Autodesk Fusion 360 part; units mm, degrees
(part 4 of 6)
  line L1889 (94.173, 59.875) -> (98.4623, 59.875)
  line L1890 (93.1162, 65.9119) -> (93.971, 59.875)
  line L1891 (98.4284, 66.8385) -> (97.7686, 66.2013)
  line L1892 (93.9606, 61.375) -> (94.173, 59.875)
  line L1893 (93.1277, 66.1876) -> (97.4664, 66.1876)
  line L1894 (98.4003, 67.0365) -> (97.5043, 67.9621)
  line L1895 (91.4702, 66.8375) -> (92.2202, 66.8375)
  line L1896 (99.1784, 66.8385) -> (98.4284, 66.8385)
  arc A278 (92.3951, 60.3049) -> (92.8902, 59.875) centre (92.8902, 60.375) ccw
  line L1897 (92.1918, 67.0375) -> (91.4418, 67.0375)
  line L1898 (96.4494, 74) -> (96.6618, 72.5)
  arc A279 (98.2252, 73.5701) -> (97.7301, 74) centre (97.7301, 73.5) ccw
  line L1899 (91.4418, 67.0375) -> (90.456, 74)
  line L1900 (92.3834, 72.5) -> (92.171, 74)
  line L1901 (98.1643, 74) -> (99.1503, 67.0365)
  line L1902 (92.3894, 66.9502) -> (93.1277, 66.1876)
  line L1903 (91.971, 74) -> (92.8648, 67.6874)
  line L1904 (98.23, 66.9249) -> (97.4917, 67.6876)
  line L1905 (97.5043, 67.9621) -> (96.6494, 74)
  line L1906 (92.171, 74) -> (96.4494, 74)
  line L1907 (97.4917, 67.6876) -> (93.1529, 67.6876)
  line L1908 (96.6494, 74) -> (98.1643, 74)
  line L1909 (92.8648, 67.6874) -> (92.1918, 67.0375)
  line L1910 (109.3698, 72.5) -> (105.0914, 72.5)
  line L1911 (104.679, 74) -> (103.164, 74)
  arc A280 (112.2965, 59.875) -> (112.7916, 60.4451) centre (112.2965, 60.375) ccw
  circle A281 centre (103.164, 60.75) radius 0.875
  line L1912 (104.9282, 66.8375) -> (105.8242, 65.9119)
  line L1913 (111.3723, 59.875) -> (112.8723, 59.875)
  line L1914 (110.9579, 61.375) -> (106.6686, 61.375)
  line L1915 (105.8609, 67.6876) -> (105.0974, 66.9502)
  line L1916 (106.679, 59.875) -> (105.164, 59.875)
  line L1917 (105.164, 59.875) -> (104.1782, 66.8375)
  line L1918 (110.4766, 66.2013) -> (111.3723, 59.875)
  line L1919 (111.1703, 59.875) -> (110.9579, 61.375)
  line L1920 (110.1744, 66.1876) -> (110.938, 66.9249)
  line L1921 (111.8583, 67.0365) -> (111.1083, 67.0365)
  line L1922 (112.8723, 59.875) -> (111.8864, 66.8385)
  arc A282 (103.7398, 74) -> (103.2447, 73.4299) centre (103.7398, 73.5) ccw
  line L1923 (106.881, 59.875) -> (111.1703, 59.875)
  line L1924 (105.8242, 65.9119) -> (106.679, 59.875)
  line L1925 (111.1364, 66.8385) -> (110.4766, 66.2013)
  line L1926 (106.6686, 61.375) -> (106.881, 59.875)
  line L1927 (105.8357, 66.1876) -> (110.1744, 66.1876)
  line L1928 (111.1083, 67.0365) -> (110.2123, 67.9621)
  line L1929 (104.1782, 66.8375) -> (104.9282, 66.8375)
  line L1930 (111.8864, 66.8385) -> (111.1364, 66.8385)
  arc A283 (105.1031, 60.3049) -> (105.5982, 59.875) centre (105.5982, 60.375) ccw
  line L1931 (104.8998, 67.0375) -> (104.1498, 67.0375)
  line L1932 (109.1574, 74) -> (109.3698, 72.5)
  arc A284 (110.9332, 73.5701) -> (110.4381, 74) centre (110.4381, 73.5) ccw
  line L1933 (104.1498, 67.0375) -> (103.164, 74)
  line L1934 (105.0914, 72.5) -> (104.879, 74)
  line L1935 (110.8723, 74) -> (111.8583, 67.0365)
  line L1936 (105.0974, 66.9502) -> (105.8357, 66.1876)
  line L1937 (104.679, 74) -> (105.5728, 67.6874)
  line L1938 (110.938, 66.9249) -> (110.1997, 67.6876)
  line L1939 (110.2123, 67.9621) -> (109.3574, 74)
  line L1940 (104.879, 74) -> (109.1574, 74)
  line L1941 (110.1997, 67.6876) -> (105.8609, 67.6876)
  line L1942 (109.3574, 74) -> (110.8723, 74)
  line L1943 (105.5728, 67.6874) -> (104.8998, 67.0375)
  line L1944 (122.0778, 72.5) -> (117.7994, 72.5)
  line L1945 (117.387, 74) -> (115.872, 74)
  arc A285 (125.0045, 59.875) -> (125.4996, 60.4451) centre (125.0045, 60.375) ccw
  circle A286 centre (115.872, 60.75) radius 0.875
  line L1946 (117.6362, 66.8375) -> (118.5322, 65.9119)
  line L1947 (124.0803, 59.875) -> (125.5803, 59.875)
  line L1948 (123.6659, 61.375) -> (119.3766, 61.375)
  line L1949 (118.5689, 67.6876) -> (117.8054, 66.9502)
  line L1950 (119.387, 59.875) -> (117.872, 59.875)
  line L1951 (117.872, 59.875) -> (116.8862, 66.8375)
  line L1952 (123.1846, 66.2013) -> (124.0803, 59.875)
  line L1953 (123.8783, 59.875) -> (123.6659, 61.375)
  line L1954 (122.8824, 66.1876) -> (123.646, 66.9249)
  line L1955 (124.5663, 67.0365) -> (123.8163, 67.0365)
  line L1956 (125.5803, 59.875) -> (124.5944, 66.8385)
  arc A287 (116.4478, 74) -> (115.9527, 73.4299) centre (116.4478, 73.5) ccw
  line L1957 (119.589, 59.875) -> (123.8783, 59.875)
  line L1958 (118.5322, 65.9119) -> (119.387, 59.875)
  line L1959 (123.8444, 66.8385) -> (123.1846, 66.2013)
  line L1960 (119.3766, 61.375) -> (119.589, 59.875)
  line L1961 (118.5437, 66.1876) -> (122.8824, 66.1876)
  line L1962 (123.8163, 67.0365) -> (122.9203, 67.9621)
  line L1963 (116.8862, 66.8375) -> (117.6362, 66.8375)
  line L1964 (124.5944, 66.8385) -> (123.8444, 66.8385)
  arc A288 (117.8111, 60.3049) -> (118.3062, 59.875) centre (118.3062, 60.375) ccw
  line L1965 (117.6078, 67.0375) -> (116.8578, 67.0375)
  line L1966 (121.8654, 74) -> (122.0778, 72.5)
  arc A289 (123.6412, 73.5701) -> (123.1461, 74) centre (123.1461, 73.5) ccw
  line L1967 (116.8578, 67.0375) -> (115.872, 74)
  line L1968 (117.7994, 72.5) -> (117.587, 74)
  line L1969 (123.5803, 74) -> (124.5663, 67.0365)
  line L1970 (117.8054, 66.9502) -> (118.5437, 66.1876)
  line L1971 (117.387, 74) -> (118.2808, 67.6874)
  line L1972 (123.646, 66.9249) -> (122.9077, 67.6876)
  line L1973 (122.9203, 67.9621) -> (122.0654, 74)
  line L1974 (117.587, 74) -> (121.8654, 74)
  line L1975 (122.9077, 67.6876) -> (118.5689, 67.6876)
  line L1976 (122.0654, 74) -> (123.5803, 74)
  line L1977 (118.2808, 67.6874) -> (117.6078, 67.0375)
  line L1978 (134.7858, 72.5) -> (130.5074, 72.5)
  line L1979 (130.095, 74) -> (128.58, 74)
  arc A290 (137.7125, 59.875) -> (138.2076, 60.4451) centre (137.7125, 60.375) ccw
  circle A291 centre (128.58, 60.75) radius 0.875
  line L1980 (130.3442, 66.8375) -> (131.2402, 65.9119)
  line L1981 (136.7883, 59.875) -> (138.2883, 59.875)
  line L1982 (136.3739, 61.375) -> (132.0846, 61.375)
  line L1983 (131.2769, 67.6876) -> (130.5134, 66.9502)
  line L1984 (132.095, 59.875) -> (130.58, 59.875)
  line L1985 (130.58, 59.875) -> (129.5942, 66.8375)
  line L1986 (135.8926, 66.2013) -> (136.7883, 59.875)
  line L1987 (136.5863, 59.875) -> (136.3739, 61.375)
  line L1988 (135.5904, 66.1876) -> (136.354, 66.9249)
  line L1989 (137.2743, 67.0365) -> (136.5243, 67.0365)
  line L1990 (138.2883, 59.875) -> (137.3024, 66.8385)
  arc A292 (129.1558, 74) -> (128.6607, 73.4299) centre (129.1558, 73.5) ccw
  line L1991 (132.297, 59.875) -> (136.5863, 59.875)
  line L1992 (131.2402, 65.9119) -> (132.095, 59.875)
  line L1993 (136.5524, 66.8385) -> (135.8926, 66.2013)
  line L1994 (132.0846, 61.375) -> (132.297, 59.875)
  line L1995 (131.2517, 66.1876) -> (135.5904, 66.1876)
  line L1996 (136.5243, 67.0365) -> (135.6283, 67.9621)
  line L1997 (129.5942, 66.8375) -> (130.3442, 66.8375)
  line L1998 (137.3024, 66.8385) -> (136.5524, 66.8385)
  arc A293 (130.5191, 60.3049) -> (131.0142, 59.875) centre (131.0142, 60.375) ccw
  line L1999 (130.3158, 67.0375) -> (129.5658, 67.0375)
  line L2000 (134.5734, 74) -> (134.7858, 72.5)
  arc A294 (136.3492, 73.5701) -> (135.8541, 74) centre (135.8541, 73.5) ccw
  line L2001 (129.5658, 67.0375) -> (128.58, 74)
  line L2002 (130.5074, 72.5) -> (130.295, 74)
  line L2003 (136.2883, 74) -> (137.2743, 67.0365)
  line L2004 (130.5134, 66.9502) -> (131.2517, 66.1876)
  line L2005 (130.095, 74) -> (130.9888, 67.6874)
  line L2006 (136.354, 66.9249) -> (135.6157, 67.6876)
  line L2007 (135.6283, 67.9621) -> (134.7734, 74)
  line L2008 (130.295, 74) -> (134.5734, 74)
  line L2009 (135.6157, 67.6876) -> (131.2769, 67.6876)
  line L2010 (134.7734, 74) -> (136.2883, 74)
  line L2011 (130.9888, 67.6874) -> (130.3158, 67.0375)
  line L2012 (147.4938, 72.5) -> (143.2154, 72.5)
  line L2013 (142.803, 74) -> (141.288, 74)
  arc A295 (150.4205, 59.875) -> (150.9156, 60.4451) centre (150.4205, 60.375) ccw
  circle A296 centre (141.288, 60.75) radius 0.875
  line L2014 (143.0522, 66.8375) -> (143.9482, 65.9119)
  line L2015 (149.4963, 59.875) -> (150.9963, 59.875)
  line L2016 (149.0819, 61.375) -> (144.7926, 61.375)
  line L2017 (143.9849, 67.6876) -> (143.2214, 66.9502)
  line L2018 (144.803, 59.875) -> (143.288, 59.875)
  line L2019 (143.288, 59.875) -> (142.3022, 66.8375)
  line L2020 (148.6006, 66.2013) -> (149.4963, 59.875)
  line L2021 (149.2943, 59.875) -> (149.0819, 61.375)
  line L2022 (148.2984, 66.1876) -> (149.062, 66.9249)
  line L2023 (149.9823, 67.0365) -> (149.2323, 67.0365)
  line L2024 (150.9963, 59.875) -> (150.0104, 66.8385)
  arc A297 (141.8638, 74) -> (141.3687, 73.4299) centre (141.8638, 73.5) ccw
  line L2025 (145.005, 59.875) -> (149.2943, 59.875)
  line L2026 (143.9482, 65.9119) -> (144.803, 59.875)
  line L2027 (149.2604, 66.8385) -> (148.6006, 66.2013)
  line L2028 (144.7926, 61.375) -> (145.005, 59.875)
  line L2029 (143.9597, 66.1876) -> (148.2984, 66.1876)
  line L2030 (149.2323, 67.0365) -> (148.3363, 67.9621)
  line L2031 (142.3022, 66.8375) -> (143.0522, 66.8375)
  line L2032 (150.0104, 66.8385) -> (149.2604, 66.8385)
  arc A298 (143.2271, 60.3049) -> (143.7222, 59.875) centre (143.7222, 60.375) ccw
  line L2033 (143.0238, 67.0375) -> (142.2738, 67.0375)
  line L2034 (147.2814, 74) -> (147.4938, 72.5)
  arc A299 (149.0572, 73.5701) -> (148.5621, 74) centre (148.5621, 73.5) ccw
  line L2035 (142.2738, 67.0375) -> (141.288, 74)
  line L2036 (143.2154, 72.5) -> (143.003, 74)
  line L2037 (148.9963, 74) -> (149.9823, 67.0365)
  line L2038 (143.2214, 66.9502) -> (143.9597, 66.1876)
  line L2039 (142.803, 74) -> (143.6968, 67.6874)
  line L2040 (149.062, 66.9249) -> (148.3237, 67.6876)
  line L2041 (148.3363, 67.9621) -> (147.4814, 74)
  line L2042 (143.003, 74) -> (147.2814, 74)
  line L2043 (148.3237, 67.6876) -> (143.9849, 67.6876)
  line L2044 (147.4814, 74) -> (148.9963, 74)
  line L2045 (143.6968, 67.6874) -> (143.0238, 67.0375)
  line L2046 (160.2018, 72.5) -> (155.9234, 72.5)
  line L2047 (155.511, 74) -> (153.996, 74)
  arc A300 (163.1285, 59.875) -> (163.6236, 60.4451) centre (163.1285, 60.375) ccw
  circle A301 centre (153.996, 60.75) radius 0.875
  line L2048 (155.7602, 66.8375) -> (156.6562, 65.9119)
  line L2049 (162.2043, 59.875) -> (163.7043, 59.875)
  line L2050 (161.7899, 61.375) -> (157.5006, 61.375)
  line L2051 (156.6929, 67.6876) -> (155.9294, 66.9502)
  line L2052 (157.511, 59.875) -> (155.996, 59.875)
  line L2053 (155.996, 59.875) -> (155.0102, 66.8375)
  line L2054 (161.3086, 66.2013) -> (162.2043, 59.875)
  line L2055 (162.0023, 59.875) -> (161.7899, 61.375)
  line L2056 (161.0064, 66.1876) -> (161.77, 66.9249)
  line L2057 (162.6903, 67.0365) -> (161.9403, 67.0365)
  line L2058 (163.7043, 59.875) -> (162.7184, 66.8385)
  arc A302 (154.5718, 74) -> (154.0767, 73.4299) centre (154.5718, 73.5) ccw
  line L2059 (157.713, 59.875) -> (162.0023, 59.875)
  line L2060 (156.6562, 65.9119) -> (157.511, 59.875)
  line L2061 (161.9684, 66.8385) -> (161.3086, 66.2013)
  line L2062 (157.5006, 61.375) -> (157.713, 59.875)
  line L2063 (156.6677, 66.1876) -> (161.0064, 66.1876)
  line L2064 (161.9403, 67.0365) -> (161.0443, 67.9621)
  line L2065 (155.0102, 66.8375) -> (155.7602, 66.8375)
  line L2066 (162.7184, 66.8385) -> (161.9684, 66.8385)
  arc A303 (155.9351, 60.3049) -> (156.4302, 59.875) centre (156.4302, 60.375) ccw
  line L2067 (155.7318, 67.0375) -> (154.9818, 67.0375)
  line L2068 (159.9894, 74) -> (160.2018, 72.5)
  arc A304 (161.7652, 73.5701) -> (161.2701, 74) centre (161.2701, 73.5) ccw
  line L2069 (154.9818, 67.0375) -> (153.996, 74)
  line L2070 (155.9234, 72.5) -> (155.711, 74)
  line L2071 (161.7043, 74) -> (162.6903, 67.0365)
  line L2072 (155.9294, 66.9502) -> (156.6677, 66.1876)
  line L2073 (155.511, 74) -> (156.4048, 67.6874)
  line L2074 (161.77, 66.9249) -> (161.0317, 67.6876)
  line L2075 (161.0443, 67.9621) -> (160.1894, 74)
  line L2076 (155.711, 74) -> (159.9894, 74)
  line L2077 (161.0317, 67.6876) -> (156.6929, 67.6876)
  line L2078 (160.1894, 74) -> (161.7043, 74)
  line L2079 (156.4048, 67.6874) -> (155.7318, 67.0375)
  line L2080 (172.9098, 72.5) -> (168.6314, 72.5)
  line L2081 (168.219, 74) -> (166.704, 74)
  arc A305 (175.8365, 59.875) -> (176.3316, 60.4451) centre (175.8365, 60.375) ccw
  circle A306 centre (166.704, 60.75) radius 0.875
  line L2082 (168.4682, 66.8375) -> (169.3642, 65.9119)
  line L2083 (174.9123, 59.875) -> (176.4123, 59.875)
  line L2084 (174.4979, 61.375) -> (170.2086, 61.375)
  line L2085 (169.4009, 67.6876) -> (168.6374, 66.9502)
  line L2086 (170.219, 59.875) -> (168.704, 59.875)
  line L2087 (168.704, 59.875) -> (167.7182, 66.8375)
  line L2088 (174.0166, 66.2013) -> (174.9123, 59.875)
  line L2089 (174.7103, 59.875) -> (174.4979, 61.375)
  line L2090 (173.7144, 66.1876) -> (174.478, 66.9249)
  line L2091 (175.3983, 67.0365) -> (174.6483, 67.0365)
  line L2092 (176.4123, 59.875) -> (175.4264, 66.8385)
  arc A307 (167.2798, 74) -> (166.7847, 73.4299) centre (167.2798, 73.5) ccw
  line L2093 (170.421, 59.875) -> (174.7103, 59.875)
  line L2094 (169.3642, 65.9119) -> (170.219, 59.875)
  line L2095 (174.6764, 66.8385) -> (174.0166, 66.2013)
  line L2096 (170.2086, 61.375) -> (170.421, 59.875)
  line L2097 (169.3757, 66.1876) -> (173.7144, 66.1876)
  line L2098 (174.6483, 67.0365) -> (173.7523, 67.9621)
  line L2099 (167.7182, 66.8375) -> (168.4682, 66.8375)
  line L2100 (175.4264, 66.8385) -> (174.6764, 66.8385)
  arc A308 (168.6431, 60.3049) -> (169.1382, 59.875) centre (169.1382, 60.375) ccw
  line L2101 (168.4398, 67.0375) -> (167.6898, 67.0375)
  line L2102 (172.6974, 74) -> (172.9098, 72.5)
  arc A309 (174.4732, 73.5701) -> (173.9781, 74) centre (173.9781, 73.5) ccw
  line L2103 (167.6898, 67.0375) -> (166.704, 74)
  line L2104 (168.6314, 72.5) -> (168.419, 74)
  line L2105 (174.4123, 74) -> (175.3983, 67.0365)
  line L2106 (168.6374, 66.9502) -> (169.3757, 66.1876)
  line L2107 (168.219, 74) -> (169.1128, 67.6874)
  line L2108 (174.478, 66.9249) -> (173.7397, 67.6876)
  line L2109 (173.7523, 67.9621) -> (172.8974, 74)
  line L2110 (168.419, 74) -> (172.6974, 74)
  line L2111 (173.7397, 67.6876) -> (169.4009, 67.6876)
  line L2112 (172.8974, 74) -> (174.4123, 74)
  line L2113 (169.1128, 67.6874) -> (168.4398, 67.0375)
  line L2114 (185.6178, 72.5) -> (181.3394, 72.5)
  line L2115 (180.927, 74) -> (179.412, 74)
  arc A310 (188.5445, 59.875) -> (189.0396, 60.4451) centre (188.5445, 60.375) ccw
  circle A311 centre (179.412, 60.75) radius 0.875
  line L2116 (181.1762, 66.8375) -> (182.0722, 65.9119)
  line L2117 (187.6203, 59.875) -> (189.1203, 59.875)
  line L2118 (187.2059, 61.375) -> (182.9166, 61.375)
  line L2119 (182.1089, 67.6876) -> (181.3454, 66.9502)
  line L2120 (182.927, 59.875) -> (181.412, 59.875)
  line L2121 (181.412, 59.875) -> (180.4262, 66.8375)
  line L2122 (186.7246, 66.2013) -> (187.6203, 59.875)
  line L2123 (187.4183, 59.875) -> (187.2059, 61.375)
  line L2124 (186.4224, 66.1876) -> (187.186, 66.9249)
  line L2125 (188.1063, 67.0365) -> (187.3563, 67.0365)
  line L2126 (189.1203, 59.875) -> (188.1344, 66.8385)
  arc A312 (179.9878, 74) -> (179.4927, 73.4299) centre (179.9878, 73.5) ccw
  line L2127 (183.129, 59.875) -> (187.4183, 59.875)
  line L2128 (182.0722, 65.9119) -> (182.927, 59.875)
  line L2129 (187.3844, 66.8385) -> (186.7246, 66.2013)
  line L2130 (182.9166, 61.375) -> (183.129, 59.875)
  line L2131 (182.0837, 66.1876) -> (186.4224, 66.1876)
  line L2132 (187.3563, 67.0365) -> (186.4603, 67.9621)
  line L2133 (180.4262, 66.8375) -> (181.1762, 66.8375)
  line L2134 (188.1344, 66.8385) -> (187.3844, 66.8385)
  arc A313 (181.3511, 60.3049) -> (181.8462, 59.875) centre (181.8462, 60.375) ccw
  line L2135 (181.1478, 67.0375) -> (180.3978, 67.0375)
  line L2136 (185.4054, 74) -> (185.6178, 72.5)
  arc A314 (187.1812, 73.5701) -> (186.6861, 74) centre (186.6861, 73.5) ccw
  line L2137 (180.3978, 67.0375) -> (179.412, 74)
  line L2138 (181.3394, 72.5) -> (181.127, 74)
  line L2139 (187.1203, 74) -> (188.1063, 67.0365)
  line L2140 (181.3454, 66.9502) -> (182.0837, 66.1876)
  line L2141 (180.927, 74) -> (181.8208, 67.6874)
  line L2142 (187.186, 66.9249) -> (186.4477, 67.6876)
  line L2143 (186.4603, 67.9621) -> (185.6054, 74)
  line L2144 (181.127, 74) -> (185.4054, 74)
  line L2145 (186.4477, 67.6876) -> (182.1089, 67.6876)
  line L2146 (185.6054, 74) -> (187.1203, 74)
  line L2147 (181.8208, 67.6874) -> (181.1478, 67.0375)
  line L2148 (198.3258, 72.5) -> (194.0474, 72.5)
  line L2149 (193.635, 74) -> (192.12, 74)
  arc A315 (201.2525, 59.875) -> (201.7476, 60.4451) centre (201.2525, 60.375) ccw
  circle A316 centre (192.12, 60.75) radius 0.875
  line L2150 (193.8842, 66.8375) -> (194.7802, 65.9119)
  line L2151 (200.3283, 59.875) -> (201.8283, 59.875)
  line L2152 (199.9139, 61.375) -> (195.6246, 61.375)
  line L2153 (194.8169, 67.6876) -> (194.0534, 66.9502)
  line L2154 (195.635, 59.875) -> (194.12, 59.875)
  line L2155 (194.12, 59.875) -> (193.1342, 66.8375)
  line L2156 (199.4326, 66.2013) -> (200.3283, 59.875)
  line L2157 (200.1263, 59.875) -> (199.9139, 61.375)
  line L2158 (199.1304, 66.1876) -> (199.894, 66.9249)
  line L2159 (200.8143, 67.0365) -> (200.0643, 67.0365)
  line L2160 (201.8283, 59.875) -> (200.8424, 66.8385)
  arc A317 (192.6958, 74) -> (192.2007, 73.4299) centre (192.6958, 73.5) ccw
  line L2161 (195.837, 59.875) -> (200.1263, 59.875)
  line L2162 (194.7802, 65.9119) -> (195.635, 59.875)
  line L2163 (200.0924, 66.8385) -> (199.4326, 66.2013)
  line L2164 (195.6246, 61.375) -> (195.837, 59.875)
  line L2165 (194.7917, 66.1876) -> (199.1304, 66.1876)
  line L2166 (200.0643, 67.0365) -> (199.1683, 67.9621)
  line L2167 (193.1342, 66.8375) -> (193.8842, 66.8375)
  line L2168 (200.8424, 66.8385) -> (200.0924, 66.8385)
  arc A318 (194.0591, 60.3049) -> (194.5542, 59.875) centre (194.5542, 60.375) ccw
  line L2169 (193.8558, 67.0375) -> (193.1058, 67.0375)
  line L2170 (198.1134, 74) -> (198.3258, 72.5)
  arc A319 (199.8892, 73.5701) -> (199.3941, 74) centre (199.3941, 73.5) ccw
  line L2171 (193.1058, 67.0375) -> (192.12, 74)
  line L2172 (194.0474, 72.5) -> (193.835, 74)
  line L2173 (199.8283, 74) -> (200.8143, 67.0365)
  line L2174 (194.0534, 66.9502) -> (194.7917, 66.1876)
  line L2175 (193.635, 74) -> (194.5288, 67.6874)
  line L2176 (199.894, 66.9249) -> (199.1557, 67.6876)
  line L2177 (199.1683, 67.9621) -> (198.3134, 74)
  line L2178 (193.835, 74) -> (198.1134, 74)
  line L2179 (199.1557, 67.6876) -> (194.8169, 67.6876)
  line L2180 (198.3134, 74) -> (199.8283, 74)
  line L2181 (194.5288, 67.6874) -> (193.8558, 67.0375)
  line L2182 (7.7058, 91.625) -> (3.4274, 91.625)
  line L2183 (3.015, 93.125) -> (1.5, 93.125)
  arc A320 (10.6325, 79) -> (11.1276, 79.5701) centre (10.6325, 79.5) ccw
  circle A321 centre (1.5, 79.875) radius 0.875
  line L2184 (3.2642, 85.9625) -> (4.1602, 85.0369)
  line L2185 (9.7083, 79) -> (11.2083, 79)
  line L2186 (9.2939, 80.5) -> (5.0046, 80.5)
  line L2187 (4.1969, 86.8126) -> (3.4334, 86.0752)
  line L2188 (5.015, 79) -> (3.5, 79)
  line L2189 (3.5, 79) -> (2.5142, 85.9625)
  line L2190 (8.8126, 85.3263) -> (9.7083, 79)
  line L2191 (9.5063, 79) -> (9.2939, 80.5)
  line L2192 (8.5104, 85.3126) -> (9.274, 86.0499)
  line L2193 (10.1943, 86.1615) -> (9.4443, 86.1615)
  line L2194 (11.2083, 79) -> (10.2224, 85.9635)
  arc A322 (2.0758, 93.125) -> (1.5807, 92.5549) centre (2.0758, 92.625) ccw
  line L2195 (5.217, 79) -> (9.5063, 79)
  line L2196 (4.1602, 85.0369) -> (5.015, 79)
  line L2197 (9.4724, 85.9635) -> (8.8126, 85.3263)
  line L2198 (5.0046, 80.5) -> (5.217, 79)
  line L2199 (4.1717, 85.3126) -> (8.5104, 85.3126)
  line L2200 (9.4443, 86.1615) -> (8.5483, 87.0871)
  line L2201 (2.5142, 85.9625) -> (3.2642, 85.9625)
  line L2202 (10.2224, 85.9635) -> (9.4724, 85.9635)
  arc A323 (3.4391, 79.4299) -> (3.9342, 79) centre (3.9342, 79.5) ccw
  line L2203 (3.2358, 86.1625) -> (2.4858, 86.1625)
  line L2204 (7.4934, 93.125) -> (7.7058, 91.625)
  arc A324 (9.2692, 92.6951) -> (8.7741, 93.125) centre (8.7741, 92.625) ccw
  line L2205 (2.4858, 86.1625) -> (1.5, 93.125)
  line L2206 (3.4274, 91.625) -> (3.215, 93.125)
  line L2207 (9.2083, 93.125) -> (10.1943, 86.1615)
  line L2208 (3.4334, 86.0752) -> (4.1717, 85.3126)
  line L2209 (3.015, 93.125) -> (3.9088, 86.8124)
  line L2210 (9.274, 86.0499) -> (8.5357, 86.8126)
  line L2211 (8.5483, 87.0871) -> (7.6934, 93.125)
  line L2212 (3.215, 93.125) -> (7.4934, 93.125)
  line L2213 (8.5357, 86.8126) -> (4.1969, 86.8126)
  line L2214 (7.6934, 93.125) -> (9.2083, 93.125)
  line L2215 (3.9088, 86.8124) -> (3.2358, 86.1625)
  line L2216 (20.4138, 91.625) -> (16.1354, 91.625)
  line L2217 (15.723, 93.125) -> (14.208, 93.125)
  arc A325 (23.3405, 79) -> (23.8356, 79.5701) centre (23.3405, 79.5) ccw
  circle A326 centre (14.208, 79.875) radius 0.875
  line L2218 (15.9722, 85.9625) -> (16.8682, 85.0369)
  line L2219 (22.4163, 79) -> (23.9163, 79)
  line L2220 (22.0019, 80.5) -> (17.7126, 80.5)
  line L2221 (16.9049, 86.8126) -> (16.1414, 86.0752)
  line L2222 (17.723, 79) -> (16.208, 79)
  line L2223 (16.208, 79) -> (15.2222, 85.9625)
  line L2224 (21.5206, 85.3263) -> (22.4163, 79)
  line L2225 (22.2143, 79) -> (22.0019, 80.5)
  line L2226 (21.2184, 85.3126) -> (21.982, 86.0499)
  line L2227 (22.9023, 86.1615) -> (22.1523, 86.1615)
  line L2228 (23.9163, 79) -> (22.9304, 85.9635)
  arc A327 (14.7838, 93.125) -> (14.2887, 92.5549) centre (14.7838, 92.625) ccw
  line L2229 (17.925, 79) -> (22.2143, 79)
  line L2230 (16.8682, 85.0369) -> (17.723, 79)
  line L2231 (22.1804, 85.9635) -> (21.5206, 85.3263)
  line L2232 (17.7126, 80.5) -> (17.925, 79)
  line L2233 (16.8797, 85.3126) -> (21.2184, 85.3126)
  line L2234 (22.1523, 86.1615) -> (21.2563, 87.0871)
  line L2235 (15.2222, 85.9625) -> (15.9722, 85.9625)
  line L2236 (22.9304, 85.9635) -> (22.1804, 85.9635)
  arc A328 (16.1471, 79.4299) -> (16.6422, 79) centre (16.6422, 79.5) ccw
  line L2237 (15.9438, 86.1625) -> (15.1938, 86.1625)
  line L2238 (20.2014, 93.125) -> (20.4138, 91.625)
  arc A329 (21.9772, 92.6951) -> (21.4821, 93.125) centre (21.4821, 92.625) ccw
  line L2239 (15.1938, 86.1625) -> (14.208, 93.125)
  line L2240 (16.1354, 91.625) -> (15.923, 93.125)
  line L2241 (21.9163, 93.125) -> (22.9023, 86.1615)
  line L2242 (16.1414, 86.0752) -> (16.8797, 85.3126)
  line L2243 (15.723, 93.125) -> (16.6168, 86.8124)
  line L2244 (21.982, 86.0499) -> (21.2437, 86.8126)
  line L2245 (21.2563, 87.0871) -> (20.4014, 93.125)
  line L2246 (15.923, 93.125) -> (20.2014, 93.125)
  line L2247 (21.2437, 86.8126) -> (16.9049, 86.8126)
  line L2248 (20.4014, 93.125) -> (21.9163, 93.125)
  line L2249 (16.6168, 86.8124) -> (15.9438, 86.1625)
  line L2250 (33.1218, 91.625) -> (28.8434, 91.625)
  line L2251 (28.431, 93.125) -> (26.916, 93.125)
  arc A330 (36.0485, 79) -> (36.5436, 79.5701) centre (36.0485, 79.5) ccw
  circle A331 centre (26.916, 79.875) radius 0.875
  line L2252 (28.6802, 85.9625) -> (29.5762, 85.0369)
  line L2253 (35.1243, 79) -> (36.6243, 79)
  line L2254 (34.7099, 80.5) -> (30.4206, 80.5)
  line L2255 (29.6129, 86.8126) -> (28.8494, 86.0752)
  line L2256 (30.431, 79) -> (28.916, 79)
  line L2257 (28.916, 79) -> (27.9302, 85.9625)
  line L2258 (34.2286, 85.3263) -> (35.1243, 79)
  line L2259 (34.9223, 79) -> (34.7099, 80.5)
  line L2260 (33.9264, 85.3126) -> (34.69, 86.0499)
  line L2261 (35.6103, 86.1615) -> (34.8603, 86.1615)
  line L2262 (36.6243, 79) -> (35.6384, 85.9635)
  arc A332 (27.4918, 93.125) -> (26.9967, 92.5549) centre (27.4918, 92.625) ccw
  line L2263 (30.633, 79) -> (34.9223, 79)
  line L2264 (29.5762, 85.0369) -> (30.431, 79)
  line L2265 (34.8884, 85.9635) -> (34.2286, 85.3263)
  line L2266 (30.4206, 80.5) -> (30.633, 79)
  line L2267 (29.5877, 85.3126) -> (33.9264, 85.3126)
  line L2268 (34.8603, 86.1615) -> (33.9643, 87.0871)
  line L2269 (27.9302, 85.9625) -> (28.6802, 85.9625)
  line L2270 (35.6384, 85.9635) -> (34.8884, 85.9635)
  arc A333 (28.8551, 79.4299) -> (29.3502, 79) centre (29.3502, 79.5) ccw
  line L2271 (28.6518, 86.1625) -> (27.9018, 86.1625)
  line L2272 (32.9094, 93.125) -> (33.1218, 91.625)
  arc A334 (34.6852, 92.6951) -> (34.1901, 93.125) centre (34.1901, 92.625) ccw
  line L2273 (27.9018, 86.1625) -> (26.916, 93.125)
  line L2274 (28.8434, 91.625) -> (28.631, 93.125)
  line L2275 (34.6243, 93.125) -> (35.6103, 86.1615)
  line L2276 (28.8494, 86.0752) -> (29.5877, 85.3126)
  line L2277 (28.431, 93.125) -> (29.3248, 86.8124)
  line L2278 (34.69, 86.0499) -> (33.9517, 86.8126)
  line L2279 (33.9643, 87.0871) -> (33.1094, 93.125)
  line L2280 (28.631, 93.125) -> (32.9094, 93.125)
  line L2281 (33.9517, 86.8126) -> (29.6129, 86.8126)
  line L2282 (33.1094, 93.125) -> (34.6243, 93.125)
  line L2283 (29.3248, 86.8124) -> (28.6518, 86.1625)
  line L2284 (45.8298, 91.625) -> (41.5514, 91.625)
  line L2285 (41.139, 93.125) -> (39.624, 93.125)
  arc A335 (48.7565, 79) -> (49.2516, 79.5701) centre (48.7565, 79.5) ccw
  circle A336 centre (39.624, 79.875) radius 0.875
  line L2286 (41.3882, 85.9625) -> (42.2842, 85.0369)
  line L2287 (47.8323, 79) -> (49.3323, 79)
  line L2288 (47.4179, 80.5) -> (43.1286, 80.5)
  line L2289 (42.3209, 86.8126) -> (41.5574, 86.0752)
  line L2290 (43.139, 79) -> (41.624, 79)
  line L2291 (41.624, 79) -> (40.6382, 85.9625)
  line L2292 (46.9366, 85.3263) -> (47.8323, 79)
  line L2293 (47.6303, 79) -> (47.4179, 80.5)
  line L2294 (46.6344, 85.3126) -> (47.398, 86.0499)
  line L2295 (48.3183, 86.1615) -> (47.5683, 86.1615)
  line L2296 (49.3323, 79) -> (48.3464, 85.9635)
  arc A337 (40.1998, 93.125) -> (39.7047, 92.5549) centre (40.1998, 92.625) ccw
  line L2297 (43.341, 79) -> (47.6303, 79)
  line L2298 (42.2842, 85.0369) -> (43.139, 79)
  line L2299 (47.5964, 85.9635) -> (46.9366, 85.3263)
  line L2300 (43.1286, 80.5) -> (43.341, 79)
  line L2301 (42.2957, 85.3126) -> (46.6344, 85.3126)
  line L2302 (47.5683, 86.1615) -> (46.6723, 87.0871)
  line L2303 (40.6382, 85.9625) -> (41.3882, 85.9625)
  line L2304 (48.3464, 85.9635) -> (47.5964, 85.9635)
  arc A338 (41.5631, 79.4299) -> (42.0582, 79) centre (42.0582, 79.5) ccw
  line L2305 (41.3598, 86.1625) -> (40.6098, 86.1625)
  line L2306 (45.6174, 93.125) -> (45.8298, 91.625)
  arc A339 (47.3932, 92.6951) -> (46.8981, 93.125) centre (46.8981, 92.625) ccw
  line L2307 (40.6098, 86.1625) -> (39.624, 93.125)
  line L2308 (41.5514, 91.625) -> (41.339, 93.125)
  line L2309 (47.3323, 93.125) -> (48.3183, 86.1615)
  line L2310 (41.5574, 86.0752) -> (42.2957, 85.3126)
  line L2311 (41.139, 93.125) -> (42.0328, 86.8124)
  line L2312 (47.398, 86.0499) -> (46.6597, 86.8126)
  line L2313 (46.6723, 87.0871) -> (45.8174, 93.125)
  line L2314 (41.339, 93.125) -> (45.6174, 93.125)
  line L2315 (46.6597, 86.8126) -> (42.3209, 86.8126)
  line L2316 (45.8174, 93.125) -> (47.3323, 93.125)
  line L2317 (42.0328, 86.8124) -> (41.3598, 86.1625)
  line L2318 (58.5378, 91.625) -> (54.2594, 91.625)
  line L2319 (53.847, 93.125) -> (52.332, 93.125)
  arc A340 (61.4645, 79) -> (61.9596, 79.5701) centre (61.4645, 79.5) ccw
  circle A341 centre (52.332, 79.875) radius 0.875
  line L2320 (54.0962, 85.9625) -> (54.9922, 85.0369)
  line L2321 (60.5403, 79) -> (62.0403, 79)
  line L2322 (60.1259, 80.5) -> (55.8366, 80.5)
  line L2323 (55.0289, 86.8126) -> (54.2654, 86.0752)
  line L2324 (55.847, 79) -> (54.332, 79)
  line L2325 (54.332, 79) -> (53.3462, 85.9625)
  line L2326 (59.6446, 85.3263) -> (60.5403, 79)
  line L2327 (60.3383, 79) -> (60.1259, 80.5)
  line L2328 (59.3424, 85.3126) -> (60.106, 86.0499)
  line L2329 (61.0263, 86.1615) -> (60.2763, 86.1615)
  line L2330 (62.0403, 79) -> (61.0544, 85.9635)
  arc A342 (52.9078, 93.125) -> (52.4127, 92.5549) centre (52.9078, 92.625) ccw
  line L2331 (56.049, 79) -> (60.3383, 79)
  line L2332 (54.9922, 85.0369) -> (55.847, 79)
  line L2333 (60.3044, 85.9635) -> (59.6446, 85.3263)
  line L2334 (55.8366, 80.5) -> (56.049, 79)
  line L2335 (55.0037, 85.3126) -> (59.3424, 85.3126)
  line L2336 (60.2763, 86.1615) -> (59.3803, 87.0871)
  line L2337 (53.3462, 85.9625) -> (54.0962, 85.9625)
  line L2338 (61.0544, 85.9635) -> (60.3044, 85.9635)
  arc A343 (54.2711, 79.4299) -> (54.7662, 79) centre (54.7662, 79.5) ccw
  line L2339 (54.0678, 86.1625) -> (53.3178, 86.1625)
  line L2340 (58.3254, 93.125) -> (58.5378, 91.625)
  arc A344 (60.1012, 92.6951) -> (59.6061, 93.125) centre (59.6061, 92.625) ccw
  line L2341 (53.3178, 86.1625) -> (52.332, 93.125)
  line L2342 (54.2594, 91.625) -> (54.047, 93.125)
  line L2343 (60.0403, 93.125) -> (61.0263, 86.1615)
  line L2344 (54.2654, 86.0752) -> (55.0037, 85.3126)
  line L2345 (53.847, 93.125) -> (54.7408, 86.8124)
  line L2346 (60.106, 86.0499) -> (59.3677, 86.8126)
  line L2347 (59.3803, 87.0871) -> (58.5254, 93.125)
  line L2348 (54.047, 93.125) -> (58.3254, 93.125)
  line L2349 (59.3677, 86.8126) -> (55.0289, 86.8126)
  line L2350 (58.5254, 93.125) -> (60.0403, 93.125)
  line L2351 (54.7408, 86.8124) -> (54.0678, 86.1625)
  line L2352 (71.2458, 91.625) -> (66.9674, 91.625)
  line L2353 (66.555, 93.125) -> (65.04, 93.125)
  arc A345 (74.1725, 79) -> (74.6676, 79.5701) centre (74.1725, 79.5) ccw
  circle A346 centre (65.04, 79.875) radius 0.875
  line L2354 (66.8042, 85.9625) -> (67.7002, 85.0369)
  line L2355 (73.2483, 79) -> (74.7483, 79)
  line L2356 (72.8339, 80.5) -> (68.5446, 80.5)
  line L2357 (67.7369, 86.8126) -> (66.9734, 86.0752)
  line L2358 (68.555, 79) -> (67.04, 79)
  line L2359 (67.04, 79) -> (66.0542, 85.9625)
  line L2360 (72.3526, 85.3263) -> (73.2483, 79)
  line L2361 (73.0463, 79) -> (72.8339, 80.5)
  line L2362 (72.0504, 85.3126) -> (72.814, 86.0499)
  line L2363 (73.7343, 86.1615) -> (72.9843, 86.1615)
  line L2364 (74.7483, 79) -> (73.7624, 85.9635)
  arc A347 (65.6158, 93.125) -> (65.1207, 92.5549) centre (65.6158, 92.625) ccw
  line L2365 (68.757, 79) -> (73.0463, 79)
  line L2366 (67.7002, 85.0369) -> (68.555, 79)
  line L2367 (73.0124, 85.9635) -> (72.3526, 85.3263)
  line L2368 (68.5446, 80.5) -> (68.757, 79)
  line L2369 (67.7117, 85.3126) -> (72.0504, 85.3126)
  line L2370 (72.9843, 86.1615) -> (72.0883, 87.0871)
  line L2371 (66.0542, 85.9625) -> (66.8042, 85.9625)
  line L2372 (73.7624, 85.9635) -> (73.0124, 85.9635)
  arc A348 (66.9791, 79.4299) -> (67.4742, 79) centre (67.4742, 79.5) ccw
  line L2373 (66.7758, 86.1625) -> (66.0258, 86.1625)
  line L2374 (71.0334, 93.125) -> (71.2458, 91.625)
  arc A349 (72.8092, 92.6951) -> (72.3141, 93.125) centre (72.3141, 92.625) ccw
  line L2375 (66.0258, 86.1625) -> (65.04, 93.125)
  line L2376 (66.9674, 91.625) -> (66.755, 93.125)
  line L2377 (72.7483, 93.125) -> (73.7343, 86.1615)
  line L2378 (66.9734, 86.0752) -> (67.7117, 85.3126)
  line L2379 (66.555, 93.125) -> (67.4488, 86.8124)
  line L2380 (72.814, 86.0499) -> (72.0757, 86.8126)
  line L2381 (72.0883, 87.0871) -> (71.2334, 93.125)
  line L2382 (66.755, 93.125) -> (71.0334, 93.125)
  line L2383 (72.0757, 86.8126) -> (67.7369, 86.8126)
  line L2384 (71.2334, 93.125) -> (72.7483, 93.125)
  line L2385 (67.4488, 86.8124) -> (66.7758, 86.1625)
  line L2386 (83.9538, 91.625) -> (79.6754, 91.625)
  line L2387 (79.263, 93.125) -> (77.748, 93.125)
  arc A350 (86.8805, 79) -> (87.3756, 79.5701) centre (86.8805, 79.5) ccw
  circle A351 centre (77.748, 79.875) radius 0.875
  line L2388 (79.5122, 85.9625) -> (80.4082, 85.0369)
  line L2389 (85.9563, 79) -> (87.4563, 79)
  line L2390 (85.5419, 80.5) -> (81.2526, 80.5)
  line L2391 (80.4449, 86.8126) -> (79.6814, 86.0752)
  line L2392 (81.263, 79) -> (79.748, 79)
  line L2393 (79.748, 79) -> (78.7622, 85.9625)
  line L2394 (85.0606, 85.3263) -> (85.9563, 79)
  line L2395 (85.7543, 79) -> (85.5419, 80.5)
  line L2396 (84.7584, 85.3126) -> (85.522, 86.0499)
  line L2397 (86.4423, 86.1615) -> (85.6923, 86.1615)
  line L2398 (87.4563, 79) -> (86.4704, 85.9635)
  arc A352 (78.3238, 93.125) -> (77.8287, 92.5549) centre (78.3238, 92.625) ccw
  line L2399 (81.465, 79) -> (85.7543, 79)
  line L2400 (80.4082, 85.0369) -> (81.263, 79)
  line L2401 (85.7204, 85.9635) -> (85.0606, 85.3263)
  line L2402 (81.2526, 80.5) -> (81.465, 79)
  line L2403 (80.4197, 85.3126) -> (84.7584, 85.3126)
  line L2404 (85.6923, 86.1615) -> (84.7963, 87.0871)
  line L2405 (78.7622, 85.9625) -> (79.5122, 85.9625)
  line L2406 (86.4704, 85.9635) -> (85.7204, 85.9635)
  arc A353 (79.6871, 79.4299) -> (80.1822, 79) centre (80.1822, 79.5) ccw
  line L2407 (79.4838, 86.1625) -> (78.7338, 86.1625)
  line L2408 (83.7414, 93.125) -> (83.9538, 91.625)
  arc A354 (85.5172, 92.6951) -> (85.0221, 93.125) centre (85.0221, 92.625) ccw
  line L2409 (78.7338, 86.1625) -> (77.748, 93.125)
  line L2410 (79.6754, 91.625) -> (79.463, 93.125)
  line L2411 (85.4563, 93.125) -> (86.4423, 86.1615)
  line L2412 (79.6814, 86.0752) -> (80.4197, 85.3126)
  line L2413 (79.263, 93.125) -> (80.1568, 86.8124)
  line L2414 (85.522, 86.0499) -> (84.7837, 86.8126)
  line L2415 (84.7963, 87.0871) -> (83.9414, 93.125)
  line L2416 (79.463, 93.125) -> (83.7414, 93.125)
  line L2417 (84.7837, 86.8126) -> (80.4449, 86.8126)
  line L2418 (83.9414, 93.125) -> (85.4563, 93.125)
  line L2419 (80.1568, 86.8124) -> (79.4838, 86.1625)
  line L2420 (96.6618, 91.625) -> (92.3834, 91.625)
  line L2421 (91.971, 93.125) -> (90.456, 93.125)
  arc A355 (99.5885, 79) -> (100.0836, 79.5701) centre (99.5885, 79.5) ccw
  circle A356 centre (90.456, 79.875) radius 0.875
  line L2422 (92.2202, 85.9625) -> (93.1162, 85.0369)
  line L2423 (98.6643, 79) -> (100.1643, 79)
  line L2424 (98.2499, 80.5) -> (93.9606, 80.5)
  line L2425 (93.1529, 86.8126) -> (92.3894, 86.0752)
  line L2426 (93.971, 79) -> (92.456, 79)
  line L2427 (92.456, 79) -> (91.4702, 85.9625)
  line L2428 (97.7686, 85.3263) -> (98.6643, 79)
  line L2429 (98.4623, 79) -> (98.2499, 80.5)
  line L2430 (97.4664, 85.3126) -> (98.23, 86.0499)
  line L2431 (99.1503, 86.1615) -> (98.4003, 86.1615)
  line L2432 (100.1643, 79) -> (99.1784, 85.9635)
  arc A357 (91.0318, 93.125) -> (90.5367, 92.5549) centre (91.0318, 92.625) ccw
  line L2433 (94.173, 79) -> (98.4623, 79)
  line L2434 (93.1162, 85.0369) -> (93.971, 79)
  line L2435 (98.4284, 85.9635) -> (97.7686, 85.3263)
  line L2436 (93.9606, 80.5) -> (94.173, 79)
  line L2437 (93.1277, 85.3126) -> (97.4664, 85.3126)
  line L2438 (98.4003, 86.1615) -> (97.5043, 87.0871)
  line L2439 (91.4702, 85.9625) -> (92.2202, 85.9625)
  line L2440 (99.1784, 85.9635) -> (98.4284, 85.9635)
  arc A358 (92.3951, 79.4299) -> (92.8902, 79) centre (92.8902, 79.5) ccw
  line L2441 (92.1918, 86.1625) -> (91.4418, 86.1625)
  line L2442 (96.4494, 93.125) -> (96.6618, 91.625)
  arc A359 (98.2252, 92.6951) -> (97.7301, 93.125) centre (97.7301, 92.625) ccw
  line L2443 (91.4418, 86.1625) -> (90.456, 93.125)
  line L2444 (92.3834, 91.625) -> (92.171, 93.125)
  line L2445 (98.1643, 93.125) -> (99.1503, 86.1615)
  line L2446 (92.3894, 86.0752) -> (93.1277, 85.3126)
  line L2447 (91.971, 93.125) -> (92.8648, 86.8124)
  line L2448 (98.23, 86.0499) -> (97.4917, 86.8126)
  line L2449 (97.5043, 87.0871) -> (96.6494, 93.125)
  line L2450 (92.171, 93.125) -> (96.4494, 93.125)
  line L2451 (97.4917, 86.8126) -> (93.1529, 86.8126)
  line L2452 (96.6494, 93.125) -> (98.1643, 93.125)
  line L2453 (92.8648, 86.8124) -> (92.1918, 86.1625)
  line L2454 (109.3698, 91.625) -> (105.0914, 91.625)
  line L2455 (104.679, 93.125) -> (103.164, 93.125)
  arc A360 (112.2965, 79) -> (112.7916, 79.5701) centre (112.2965, 79.5) ccw
  circle A361 centre (103.164, 79.875) radius 0.875
  line L2456 (104.9282, 85.9625) -> (105.8242, 85.0369)
  line L2457 (111.3723, 79) -> (112.8723, 79)
  line L2458 (110.9579, 80.5) -> (106.6686, 80.5)
  line L2459 (105.8609, 86.8126) -> (105.0974, 86.0752)
  line L2460 (106.679, 79) -> (105.164, 79)
  line L2461 (105.164, 79) -> (104.1782, 85.9625)
  line L2462 (110.4766, 85.3263) -> (111.3723, 79)
  line L2463 (111.1703, 79) -> (110.9579, 80.5)
  line L2464 (110.1744, 85.3126) -> (110.938, 86.0499)
  line L2465 (111.8583, 86.1615) -> (111.1083, 86.1615)
  line L2466 (112.8723, 79) -> (111.8864, 85.9635)
  arc A362 (103.7398, 93.125) -> (103.2447, 92.5549) centre (103.7398, 92.625) ccw
  line L2467 (106.881, 79) -> (111.1703, 79)
  line L2468 (105.8242, 85.0369) -> (106.679, 79)
  line L2469 (111.1364, 85.9635) -> (110.4766, 85.3263)
  line L2470 (106.6686, 80.5) -> (106.881, 79)
  line L2471 (105.8357, 85.3126) -> (110.1744, 85.3126)
  line L2472 (111.1083, 86.1615) -> (110.2123, 87.0871)
  line L2473 (104.1782, 85.9625) -> (104.9282, 85.9625)
  line L2474 (111.8864, 85.9635) -> (111.1364, 85.9635)
  arc A363 (105.1031, 79.4299) -> (105.5982, 79) centre (105.5982, 79.5) ccw
  line L2475 (104.8998, 86.1625) -> (104.1498, 86.1625)
  line L2476 (109.1574, 93.125) -> (109.3698, 91.625)
  arc A364 (110.9332, 92.6951) -> (110.4381, 93.125) centre (110.4381, 92.625) ccw
  line L2477 (104.1498, 86.1625) -> (103.164, 93.125)
  line L2478 (105.0914, 91.625) -> (104.879, 93.125)
  line L2479 (110.8723, 93.125) -> (111.8583, 86.1615)
  line L2480 (105.0974, 86.0752) -> (105.8357, 85.3126)
  line L2481 (104.679, 93.125) -> (105.5728, 86.8124)
  line L2482 (110.938, 86.0499) -> (110.1997, 86.8126)
  line L2483 (110.2123, 87.0871) -> (109.3574, 93.125)
  line L2484 (104.879, 93.125) -> (109.1574, 93.125)
  line L2485 (110.1997, 86.8126) -> (105.8609, 86.8126)
  line L2486 (109.3574, 93.125) -> (110.8723, 93.125)
  line L2487 (105.5728, 86.8124) -> (104.8998, 86.1625)
  line L2488 (122.0778, 91.625) -> (117.7994, 91.625)
  line L2489 (117.387, 93.125) -> (115.872, 93.125)
  arc A365 (125.0045, 79) -> (125.4996, 79.5701) centre (125.0045, 79.5) ccw
  circle A366 centre (115.872, 79.875) radius 0.875
  line L2490 (117.6362, 85.9625) -> (118.5322, 85.0369)
  line L2491 (124.0803, 79) -> (125.5803, 79)
  line L2492 (123.6659, 80.5) -> (119.3766, 80.5)
  line L2493 (118.5689, 86.8126) -> (117.8054, 86.0752)
  line L2494 (119.387, 79) -> (117.872, 79)
  line L2495 (117.872, 79) -> (116.8862, 85.9625)
  line L2496 (123.1846, 85.3263) -> (124.0803, 79)
  line L2497 (123.8783, 79) -> (123.6659, 80.5)
  line L2498 (122.8824, 85.3126) -> (123.646, 86.0499)
  line L2499 (124.5663, 86.1615) -> (123.8163, 86.1615)
  line L2500 (125.5803, 79) -> (124.5944, 85.9635)
  arc A367 (116.4478, 93.125) -> (115.9527, 92.5549) centre (116.4478, 92.625) ccw
  line L2501 (119.589, 79) -> (123.8783, 79)
  line L2502 (118.5322, 85.0369) -> (119.387, 79)
  line L2503 (123.8444, 85.9635) -> (123.1846, 85.3263)
  line L2504 (119.3766, 80.5) -> (119.589, 79)
  line L2505 (118.5437, 85.3126) -> (122.8824, 85.3126)
  line L2506 (123.8163, 86.1615) -> (122.9203, 87.0871)
  line L2507 (116.8862, 85.9625) -> (117.6362, 85.9625)
  line L2508 (124.5944, 85.9635) -> (123.8444, 85.9635)
  arc A368 (117.8111, 79.4299) -> (118.3062, 79) centre (118.3062, 79.5) ccw
  line L2509 (117.6078, 86.1625) -> (116.8578, 86.1625)
  line L2510 (121.8654, 93.125) -> (122.0778, 91.625)
  arc A369 (123.6412, 92.6951) -> (123.1461, 93.125) centre (123.1461, 92.625) ccw
  line L2511 (116.8578, 86.1625) -> (115.872, 93.125)
  line L2512 (117.7994, 91.625) -> (117.587, 93.125)
  line L2513 (123.5803, 93.125) -> (124.5663, 86.1615)
  line L2514 (117.8054, 86.0752) -> (118.5437, 85.3126)
  line L2515 (117.387, 93.125) -> (118.2808, 86.8124)
  line L2516 (123.646, 86.0499) -> (122.9077, 86.8126)
  line L2517 (122.9203, 87.0871) -> (122.0654, 93.125)
  line L2518 (117.587, 93.125) -> (121.8654, 93.125)
  line L2519 (122.9077, 86.8126) -> (118.5689, 86.8126)
  line L2520 (122.0654, 93.125) -> (123.5803, 93.125)
  line L2521 (118.2808, 86.8124) -> (117.6078, 86.1625)
  line L2522 (134.7858, 91.625) -> (130.5074, 91.625)
  line L2523 (130.095, 93.125) -> (128.58, 93.125)
  arc A370 (137.7125, 79) -> (138.2076, 79.5701) centre (137.7125, 79.5) ccw
  circle A371 centre (128.58, 79.875) radius 0.875
  line L2524 (130.3442, 85.9625) -> (131.2402, 85.0369)
  line L2525 (136.7883, 79) -> (138.2883, 79)
  line L2526 (136.3739, 80.5) -> (132.0846, 80.5)
  line L2527 (131.2769, 86.8126) -> (130.5134, 86.0752)
  line L2528 (132.095, 79) -> (130.58, 79)
  line L2529 (130.58, 79) -> (129.5942, 85.9625)
  line L2530 (135.8926, 85.3263) -> (136.7883, 79)
  line L2531 (136.5863, 79) -> (136.3739, 80.5)
  line L2532 (135.5904, 85.3126) -> (136.354, 86.0499)
  line L2533 (137.2743, 86.1615) -> (136.5243, 86.1615)
  line L2534 (138.2883, 79) -> (137.3024, 85.9635)
  arc A372 (129.1558, 93.125) -> (128.6607, 92.5549) centre (129.1558, 92.625) ccw
  line L2535 (132.297, 79) -> (136.5863, 79)
  line L2536 (131.2402, 85.0369) -> (132.095, 79)
  line L2537 (136.5524, 85.9635) -> (135.8926, 85.3263)
  line L2538 (132.0846, 80.5) -> (132.297, 79)
  line L2539 (131.2517, 85.3126) -> (135.5904, 85.3126)
  line L2540 (136.5243, 86.1615) -> (135.6283, 87.0871)
  line L2541 (129.5942, 85.9625) -> (130.3442, 85.9625)
  line L2542 (137.3024, 85.9635) -> (136.5524, 85.9635)
  arc A373 (130.5191, 79.4299) -> (131.0142, 79) centre (131.0142, 79.5) ccw
  line L2543 (130.3158, 86.1625) -> (129.5658, 86.1625)
  line L2544 (134.5734, 93.125) -> (134.7858, 91.625)
  arc A374 (136.3492, 92.6951) -> (135.8541, 93.125) centre (135.8541, 92.625) ccw
  line L2545 (129.5658, 86.1625) -> (128.58, 93.125)
  line L2546 (130.5074, 91.625) -> (130.295, 93.125)
  line L2547 (136.2883, 93.125) -> (137.2743, 86.1615)
  line L2548 (130.5134, 86.0752) -> (131.2517, 85.3126)
  line L2549 (130.095, 93.125) -> (130.9888, 86.8124)
  line L2550 (136.354, 86.0499) -> (135.6157, 86.8126)
  line L2551 (135.6283, 87.0871) -> (134.7734, 93.125)
  line L2552 (130.295, 93.125) -> (134.5734, 93.125)
  line L2553 (135.6157, 86.8126) -> (131.2769, 86.8126)
  line L2554 (134.7734, 93.125) -> (136.2883, 93.125)
  line L2555 (130.9888, 86.8124) -> (130.3158, 86.1625)
  line L2556 (147.4938, 91.625) -> (143.2154, 91.625)
  line L2557 (142.803, 93.125) -> (141.288, 93.125)
  arc A375 (150.4205, 79) -> (150.9156, 79.5701) centre (150.4205, 79.5) ccw
  circle A376 centre (141.288, 79.875) radius 0.875
  line L2558 (143.0522, 85.9625) -> (143.9482, 85.0369)
  line L2559 (149.4963, 79) -> (150.9963, 79)
  line L2560 (149.0819, 80.5) -> (144.7926, 80.5)
  line L2561 (143.9849, 86.8126) -> (143.2214, 86.0752)
  line L2562 (144.803, 79) -> (143.288, 79)
  line L2563 (143.288, 79) -> (142.3022, 85.9625)
  line L2564 (148.6006, 85.3263) -> (149.4963, 79)
  line L2565 (149.2943, 79) -> (149.0819, 80.5)
  line L2566 (148.2984, 85.3126) -> (149.062, 86.0499)
  line L2567 (149.9823, 86.1615) -> (149.2323, 86.1615)
  line L2568 (150.9963, 79) -> (150.0104, 85.9635)
  arc A377 (141.8638, 93.125) -> (141.3687, 92.5549) centre (141.8638, 92.625) ccw
  line L2569 (145.005, 79) -> (149.2943, 79)
  line L2570 (143.9482, 85.0369) -> (144.803, 79)
  line L2571 (149.2604, 85.9635) -> (148.6006, 85.3263)
  line L2572 (144.7926, 80.5) -> (145.005, 79)
  line L2573 (143.9597, 85.3126) -> (148.2984, 85.3126)
  line L2574 (149.2323, 86.1615) -> (148.3363, 87.0871)
  line L2575 (142.3022, 85.9625) -> (143.0522, 85.9625)
  line L2576 (150.0104, 85.9635) -> (149.2604, 85.9635)
  arc A378 (143.2271, 79.4299) -> (143.7222, 79) centre (143.7222, 79.5) ccw
  line L2577 (143.0238, 86.1625) -> (142.2738, 86.1625)
  line L2578 (147.2814, 93.125) -> (147.4938, 91.625)
  arc A379 (149.0572, 92.6951) -> (148.5621, 93.125) centre (148.5621, 92.625) ccw
  line L2579 (142.2738, 86.1625) -> (141.288, 93.125)
  line L2580 (143.2154, 91.625) -> (143.003, 93.125)
  line L2581 (148.9963, 93.125) -> (149.9823, 86.1615)
  line L2582 (143.2214, 86.0752) -> (143.9597, 85.3126)
  line L2583 (142.803, 93.125) -> (143.6968, 86.8124)
  line L2584 (149.062, 86.0499) -> (148.3237, 86.8126)
  line L2585 (148.3363, 87.0871) -> (147.4814, 93.125)
  line L2586 (143.003, 93.125) -> (147.2814, 93.125)
  line L2587 (148.3237, 86.8126) -> (143.9849, 86.8126)
  line L2588 (147.4814, 93.125) -> (148.9963, 93.125)
  line L2589 (143.6968, 86.8124) -> (143.0238, 86.1625)
  line L2590 (160.2018, 91.625) -> (155.9234, 91.625)
  line L2591 (155.511, 93.125) -> (153.996, 93.125)
  arc A380 (163.1285, 79) -> (163.6236, 79.5701) centre (163.1285, 79.5) ccw
  circle A381 centre (153.996, 79.875) radius 0.875
  line L2592 (155.7602, 85.9625) -> (156.6562, 85.0369)
  line L2593 (162.2043, 79) -> (163.7043, 79)
  line L2594 (161.7899, 80.5) -> (157.5006, 80.5)
  line L2595 (156.6929, 86.8126) -> (155.9294, 86.0752)
  line L2596 (157.511, 79) -> (155.996, 79)
  line L2597 (155.996, 79) -> (155.0102, 85.9625)
  line L2598 (161.3086, 85.3263) -> (162.2043, 79)
  line L2599 (162.0023, 79) -> (161.7899, 80.5)
  line L2600 (161.0064, 85.3126) -> (161.77, 86.0499)
  line L2601 (162.6903, 86.1615) -> (161.9403, 86.1615)
  line L2602 (163.7043, 79) -> (162.7184, 85.9635)
  arc A382 (154.5718, 93.125) -> (154.0767, 92.5549) centre (154.5718, 92.625) ccw
  line L2603 (157.713, 79) -> (162.0023, 79)
  line L2604 (156.6562, 85.0369) -> (157.511, 79)
  line L2605 (161.9684, 85.9635) -> (161.3086, 85.3263)
  line L2606 (157.5006, 80.5) -> (157.713, 79)
  line L2607 (156.6677, 85.3126) -> (161.0064, 85.3126)
  line L2608 (161.9403, 86.1615) -> (161.0443, 87.0871)
  line L2609 (155.0102, 85.9625) -> (155.7602, 85.9625)
  line L2610 (162.7184, 85.9635) -> (161.9684, 85.9635)
  arc A383 (155.9351, 79.4299) -> (156.4302, 79) centre (156.4302, 79.5) ccw
  line L2611 (155.7318, 86.1625) -> (154.9818, 86.1625)
  line L2612 (159.9894, 93.125) -> (160.2018, 91.625)
  arc A384 (161.7652, 92.6951) -> (161.2701, 93.125) centre (161.2701, 92.625) ccw
  line L2613 (154.9818, 86.1625) -> (153.996, 93.125)
  line L2614 (155.9234, 91.625) -> (155.711, 93.125)
  line L2615 (161.7043, 93.125) -> (162.6903, 86.1615)
  line L2616 (155.9294, 86.0752) -> (156.6677, 85.3126)
  line L2617 (155.511, 93.125) -> (156.4048, 86.8124)
  line L2618 (161.77, 86.0499) -> (161.0317, 86.8126)
  line L2619 (161.0443, 87.0871) -> (160.1894, 93.125)
  line L2620 (155.711, 93.125) -> (159.9894, 93.125)
  line L2621 (161.0317, 86.8126) -> (156.6929, 86.8126)
  line L2622 (160.1894, 93.125) -> (161.7043, 93.125)
  line L2623 (156.4048, 86.8124) -> (155.7318, 86.1625)
  line L2624 (172.9098, 91.625) -> (168.6314, 91.625)
  line L2625 (168.219, 93.125) -> (166.704, 93.125)
  arc A385 (175.8365, 79) -> (176.3316, 79.5701) centre (175.8365, 79.5) ccw
  circle A386 centre (166.704, 79.875) radius 0.875
  line L2626 (168.4682, 85.9625) -> (169.3642, 85.0369)
  line L2627 (174.9123, 79) -> (176.4123, 79)
  line L2628 (174.4979, 80.5) -> (170.2086, 80.5)
  line L2629 (169.4009, 86.8126) -> (168.6374, 86.0752)
  line L2630 (170.219, 79) -> (168.704, 79)
  line L2631 (168.704, 79) -> (167.7182, 85.9625)
  line L2632 (174.0166, 85.3263) -> (174.9123, 79)
  line L2633 (174.7103, 79) -> (174.4979, 80.5)
  line L2634 (173.7144, 85.3126) -> (174.478, 86.0499)
  line L2635 (175.3983, 86.1615) -> (174.6483, 86.1615)
  line L2636 (176.4123, 79) -> (175.4264, 85.9635)
  arc A387 (167.2798, 93.125) -> (166.7847, 92.5549) centre (167.2798, 92.625) ccw
  line L2637 (170.421, 79) -> (174.7103, 79)
  line L2638 (169.3642, 85.0369) -> (170.219, 79)
  line L2639 (174.6764, 85.9635) -> (174.0166, 85.3263)
  line L2640 (170.2086, 80.5) -> (170.421, 79)
  line L2641 (169.3757, 85.3126) -> (173.7144, 85.3126)
  line L2642 (174.6483, 86.1615) -> (173.7523, 87.0871)
  line L2643 (167.7182, 85.9625) -> (168.4682, 85.9625)
  line L2644 (175.4264, 85.9635) -> (174.6764, 85.9635)
  arc A388 (168.6431, 79.4299) -> (169.1382, 79) centre (169.1382, 79.5) ccw
  line L2645 (168.4398, 86.1625) -> (167.6898, 86.1625)
  line L2646 (172.6974, 93.125) -> (172.9098, 91.625)
  arc A389 (174.4732, 92.6951) -> (173.9781, 93.125) centre (173.9781, 92.625) ccw
  line L2647 (167.6898, 86.1625) -> (166.704, 93.125)
  line L2648 (168.6314, 91.625) -> (168.419, 93.125)
  line L2649 (174.4123, 93.125) -> (175.3983, 86.1615)
  line L2650 (168.6374, 86.0752) -> (169.3757, 85.3126)
  line L2651 (168.219, 93.125) -> (169.1128, 86.8124)
  line L2652 (174.478, 86.0499) -> (173.7397, 86.8126)
  line L2653 (173.7523, 87.0871) -> (172.8974, 93.125)
  line L2654 (168.419, 93.125) -> (172.6974, 93.125)
  line L2655 (173.7397, 86.8126) -> (169.4009, 86.8126)
  line L2656 (172.8974, 93.125) -> (174.4123, 93.125)
  line L2657 (169.1128, 86.8124) -> (168.4398, 86.1625)
  line L2658 (185.6178, 91.625) -> (181.3394, 91.625)
  line L2659 (180.927, 93.125) -> (179.412, 93.125)
  arc A390 (188.5445, 79) -> (189.0396, 79.5701) centre (188.5445, 79.5) ccw
  circle A391 centre (179.412, 79.875) radius 0.875
  line L2660 (181.1762, 85.9625) -> (182.0722, 85.0369)
  line L2661 (187.6203, 79) -> (189.1203, 79)
  line L2662 (187.2059, 80.5) -> (182.9166, 80.5)
  line L2663 (182.1089, 86.8126) -> (181.3454, 86.0752)
  line L2664 (182.927, 79) -> (181.412, 79)
  line L2665 (181.412, 79) -> (180.4262, 85.9625)
  line L2666 (186.7246, 85.3263) -> (187.6203, 79)
  line L2667 (187.4183, 79) -> (187.2059, 80.5)
  line L2668 (186.4224, 85.3126) -> (187.186, 86.0499)
  line L2669 (188.1063, 86.1615) -> (187.3563, 86.1615)
  line L2670 (189.1203, 79) -> (188.1344, 85.9635)
  arc A392 (179.9878, 93.125) -> (179.4927, 92.5549) centre (179.9878, 92.625) ccw
  line L2671 (183.129, 79) -> (187.4183, 79)
  line L2672 (182.0722, 85.0369) -> (182.927, 79)
  line L2673 (187.3844, 85.9635) -> (186.7246, 85.3263)
  line L2674 (182.9166, 80.5) -> (183.129, 79)
  line L2675 (182.0837, 85.3126) -> (186.4224, 85.3126)
  line L2676 (187.3563, 86.1615) -> (186.4603, 87.0871)
  line L2677 (180.4262, 85.9625) -> (181.1762, 85.9625)
  line L2678 (188.1344, 85.9635) -> (187.3844, 85.9635)
  arc A393 (181.3511, 79.4299) -> (181.8462, 79) centre (181.8462, 79.5) ccw
  line L2679 (181.1478, 86.1625) -> (180.3978, 86.1625)
  line L2680 (185.4054, 93.125) -> (185.6178, 91.625)
  arc A394 (187.1812, 92.6951) -> (186.6861, 93.125) centre (186.6861, 92.625) ccw
  line L2681 (180.3978, 86.1625) -> (179.412, 93.125)